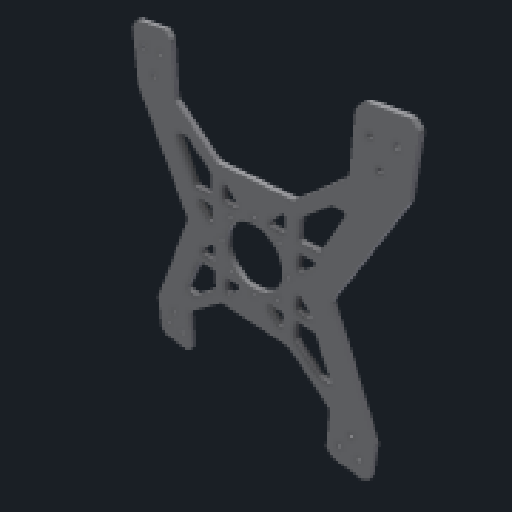
# Autodesk Inventor part: Root
Saved by Autodesk Inventor 2025.2 (Build 292293000, 293)
## iProperties
Created: 2020-05-07
Part Number: Root
Material: Generic
Document SubType Name: Sheet Metal
Designer: valer
Density: 1 g/cm^3
Sheet Metal Rule: Default
Appearance: Default
Author: valer
Autodesk Inventor part; units mm, degrees
ref_plane "YZ Plane" through (0, 0, 0) normal (1, 0, 0) x (0, 1, 0)
ref_plane "XZ Plane" through (0, 0, 0) normal (0, 1, 0) x (-1, 0, 0)
ref_plane "XY Plane" through (0, 0, 0) normal (0, 0, 1) x (1, 0, 0)
sketch "Base" plane through (0, 0, 0) normal (0, 0, 1) x (1, 0, 0)
  circle A0 centre (-56.25, 0) radius 2.75 construction
  circle A1 centre (0, -56.25) radius 2.75 construction
  circle A2 centre (0, 56.25) radius 2.75 construction
  circle A3 centre (39.7748, -39.7748) radius 2.75 construction
  circle A4 centre (-39.7748, 39.7748) radius 2.75 construction
  circle A5 centre (-39.7748, -39.7748) radius 2.75 construction
  circle A6 centre (39.7748, 39.7748) radius 2.75 construction
  circle A7 centre (56.25, 0) radius 2.75 construction
  circle A8 centre (0, 0) radius 45 construction
  circle A9 centre (0, 0) radius 61
  line L0 (-220, -170) -> (220, -170) construction
  line L1 (220, -170) -> (220, 210) construction
  line L2 (220, 210) -> (-220, 210) construction
  line L3 (-220, 210) -> (-220, -170) construction
  line L4 (0, -294) -> (0, 294) construction
  line L5 (-308, 0) -> (308, 0) construction
  line L6 (-220, 210) -> (-150, 210)
  line L7 (-150, 210) -> (-150, 130)
  line L8 (-150, 130) -> (-220, 130)
  line L9 (-220, 130) -> (-220, 210)
  line L10 (60, -103.923) -> (-60, -103.923)
  line L11 (-60, -103.923) -> (-120, 0)
  line L12 (-120, 0) -> (-60, 103.923)
  line L13 (-60, 103.923) -> (60, 103.923)
  line L14 (60, 103.923) -> (120, 0)
  line L15 (120, 0) -> (60, -103.923)
  line L16 (-120, 0) -> (-220, 130)
  line L17 (-150, 130) -> (-60, 103.923)
  line L18 (220, 210) -> (150, 210)
  line L19 (150, 210) -> (150, 130)
  line L20 (150, 130) -> (220, 130)
  line L21 (220, 130) -> (220, 210)
  line L22 (120, 0) -> (220, 130)
  line L23 (150, 130) -> (60, 103.923)
  line L24 (-220, -210) -> (-150, -210)
  line L25 (-150, -210) -> (-150, -130)
  line L26 (-150, -130) -> (-220, -170)
  line L27 (-220, -170) -> (-220, -210)
  line L28 (-120, 0) -> (-220, -170)
  line L29 (-150, -130) -> (-60, -103.923)
  line L30 (220, -170) -> (220, -210)
  line L31 (220, -210) -> (150, -210)
  line L32 (150, -210) -> (150, -130)
  line L33 (150, -130) -> (220, -170)
  line L34 (120, 0) -> (220, -170)
  line L35 (150, -130) -> (60, -103.923)
  circle A10 centre (0, 0) radius 46.5
  circle A11 centre (-56.25, 0) radius 2.25
  circle A12 centre (-39.7748, -39.7748) radius 2.25
  circle A13 centre (0, -56.25) radius 2.25
  circle A14 centre (39.7748, -39.7748) radius 2.25
  circle A15 centre (56.25, 0) radius 2.25
  circle A16 centre (39.7748, 39.7748) radius 2.25
  circle A17 centre (0, 56.25) radius 2.25
  circle A18 centre (-39.7748, 39.7748) radius 2.25
  point P0 (0, 0)
  point P1 (0, -170)
  dimension "d83" = 440
  dimension "d84" = 170
  dimension "d85" = 210
  dimension "d88" = 120
  dimension "d89" = 80
  dimension "d90" = 70
  dimension "d91" = 1.5
  dimension "d92" = 4.5
  measures "d83" distance of L0.start L0.end
  measures "d84" distance between parallel lines of L0 L5
  measures "d85" distance between parallel lines of L2 L5
  measures "d88" distance of L10.start L10.end
  measures "d89" distance between parallel lines of L2 L8
  measures "d90" distance between parallel lines of L7 L9
  measures "d91" radial gap between concentric circles of A10 A8
  measures "d92" diameter of A11
extrude "Plate1" add sketch "Base" against normal blind 8.4667 contours A9 | L6 L7 L8 L9 | L8 L17 L12 L16 | L12 L13 L14 L15 L10 L11 | L11 L29 L26 L28 | L26 L25 L24 L27 | L23 L20 L22 L14 | L15 L34 L33 L35 | L19 L18 L21 L20 | L33 L30 L31 L32
sketch "LegMountHoles" plane through (0, 0, -8.4667) normal (0, 0, -1) x (-1, 0, 0)
  line L0 (-120, 0) -> (-220, 130) construction
  line L1 (-150, 130) -> (-220, 130) construction
  line L2 (-220, 210) -> (-150, 210) construction
  line L3 (-185, 210) -> (-185, 130) construction
  line L4 (-170, 180) -> (-200, 180) construction
  circle A0 centre (-170, 180) radius 3
  circle A1 centre (-200, 180) radius 3
  circle A2 centre (-185, 150) radius 3
  line L5 (308, 0) -> (-308, 0) construction
  line L6 (0, -298) -> (0, 318) construction
  circle A3 centre (170, 180) radius 3
  circle A4 centre (200, 180) radius 3
  circle A5 centre (185, 150) radius 3
  circle A6 centre (-170, -180) radius 3
  circle A7 centre (-200, -180) radius 3
  circle A8 centre (-185, -150) radius 3
  circle A9 centre (170, -180) radius 3
  circle A10 centre (200, -180) radius 3
  circle A11 centre (185, -150) radius 3
  point P0 (0, 0)
  point P1 (-185, 180)
  dimension "d93" = 6
  dimension "d94" = 30
  dimension "d95" = 30
  dimension "d96" = 30
  constraints: 12 centre point, 9 symmetric about line, 6 end point, 3 midpoint, 2 coincident, 2 equal radius, 2 horizontal, 2 point on line, 9 other
  measures "d93" diameter of A0
  measures "d94" distance of L4.start L4.end
  measures "d95" distance from line of L4 A2.centre
  measures "d96" distance between parallel lines of L2 L4
extrude "LegMountHolesFeature" cut sketch "LegMountHoles" against normal blind 8.4667
sketch "StructureHoles" plane through (0, 0, -8.4667) normal (0, 0, -1) x (-1, 0, 0)
  line L0 (70.2991, 86.0845) -> (112.8625, 98.417)
  line L1 (112.8625, 98.417) -> (132.8625, 98.417)
  line L2 (132.8625, 98.417) -> (100.2991, 56.0845)
  line L3 (100.2991, 56.0845) -> (70.2991, 56.0845)
  line L4 (70.2991, 56.0845) -> (70.2991, 86.0845)
  line L5 (60, 103.923) -> (150, 130) projected
  line L6 (220, 130) -> (120, 0) construction
  line L7 (150, 210) -> (220, 210) projected
  line L8 (-60, 103.923) -> (60, 103.923) projected
  line L9 (60, 103.923) -> (120, 0) construction
  line L10 (50.2991, 86.0845) -> (50.2991, 56.0845)
  line L11 (50.2991, 56.0845) -> (20.2991, 56.0845)
  line L12 (20.2991, 56.0845) -> (50.2991, 86.0845)
  line L13 (70.2991, 86.0845) -> (50.2991, 86.0845) construction
  line L14 (308, 0) -> (-308, 0) construction
  line L15 (0, -298) -> (0, 318) construction
  line L16 (-70.2991, 86.0845) -> (-112.8625, 98.417)
  line L17 (-112.8625, 98.417) -> (-132.8625, 98.417)
  line L18 (-132.8625, 98.417) -> (-100.2991, 56.0845)
  line L19 (-100.2991, 56.0845) -> (-70.2991, 56.0845)
  line L20 (-70.2991, 56.0845) -> (-70.2991, 86.0845)
  line L21 (-50.2991, 86.0845) -> (-50.2991, 56.0845)
  line L22 (-50.2991, 56.0845) -> (-20.2991, 56.0845)
  line L23 (-20.2991, 56.0845) -> (-50.2991, 86.0845)
  line L24 (70.2991, -86.0845) -> (112.8625, -98.417)
  line L25 (112.8625, -98.417) -> (132.8625, -98.417)
  line L26 (132.8625, -98.417) -> (100.2991, -56.0845)
  line L27 (100.2991, -56.0845) -> (70.2991, -56.0845)
  line L28 (70.2991, -56.0845) -> (70.2991, -86.0845)
  line L29 (50.2991, -86.0845) -> (50.2991, -56.0845)
  line L30 (50.2991, -56.0845) -> (20.2991, -56.0845)
  line L31 (20.2991, -56.0845) -> (50.2991, -86.0845)
  line L32 (-132.8625, -98.417) -> (-100.2991, -56.0845)
  line L33 (-112.8625, -98.417) -> (-132.8625, -98.417)
  line L34 (-70.2991, -86.0845) -> (-112.8625, -98.417)
  line L35 (-70.2991, -56.0845) -> (-70.2991, -86.0845)
  line L36 (-100.2991, -56.0845) -> (-70.2991, -56.0845)
  line L37 (-50.2991, -86.0845) -> (-50.2991, -56.0845)
  line L38 (-20.2991, -56.0845) -> (-50.2991, -86.0845)
  line L39 (-50.2991, -56.0845) -> (-20.2991, -56.0845)
  line L40 (100.2991, 41.0845) -> (70.2991, 11.0845)
  line L41 (70.2991, 11.0845) -> (70.2991, 41.0845)
  line L42 (70.2991, 41.0845) -> (100.2991, 41.0845)
  line L43 (100.2991, 56.0845) -> (100.2991, 41.0845) construction
  line L44 (100.2991, -41.0845) -> (70.2991, -11.0845)
  line L45 (70.2991, -11.0845) -> (70.2991, -41.0845)
  line L46 (70.2991, -41.0845) -> (100.2991, -41.0845)
  line L47 (-100.2991, 41.0845) -> (-70.2991, 11.0845)
  line L48 (-70.2991, 11.0845) -> (-70.2991, 41.0845)
  line L49 (-70.2991, 41.0845) -> (-100.2991, 41.0845)
  line L50 (-100.2991, -41.0845) -> (-70.2991, -11.0845)
  line L51 (-70.2991, -41.0845) -> (-100.2991, -41.0845)
  line L52 (-70.2991, -11.0845) -> (-70.2991, -41.0845)
  point P0 (0, 0)
  point P1 (85.2991, 41.0845)
  dimension "d99" = 20
  dimension "d100" = 20
  dimension "d101" = 30
  dimension "d102" = 30
  dimension "d103" = 20
  dimension "d106" = 15
  constraints: 94 end point, 33 symmetric about line, 5 parallel, 4 perpendicular, 2 collinear, 2 equal length, 1 horizontal, 1 midpoint, 1 point on line, 1 vertical
  measures "d99" distance between parallel lines of L5 L0
  measures "d100" distance of L0.end L1.end
  measures "d101" distance of L3.end L0.start
  measures "d102" distance of L2.end L3.end
  measures "d103" distance of L0.start L10.start
  measures "d106" distance from line of point (85.299, 41.085) L3
extrude "StructureHolesFeature" cut sketch "StructureHoles" against normal blind 8.4667
fillet "InsideFilletsFeature" radius 4 44 edges at (-132.8625, 98.417, -4.2333) (-112.8625, 98.417, -4.2333) (-70.2991, 86.0845, -4.2333) (-70.2991, 56.0845, -4.2333) (-100.2991, 56.0845, -4.2333) (112.8625, 98.417, -4.2333) (132.8625, 98.417, -4.2333) (100.2991, 56.0845, -4.2333) (70.2991, 86.0845, -4.2333) (70.2991, 56.0845, -4.2333) (50.2991, 56.0845, -4.2333) (50.2991, 86.0845, -4.2333) (20.2991, 56.0845, -4.2333) (-50.2991, 86.0845, -4.2333) (-20.2991, 56.0845, -4.2333) (-50.2991, 56.0845, -4.2333) (-70.2991, 41.0845, -4.2333) (-100.2991, 41.0845, -4.2333) (-70.2991, 11.0845, -4.2333) (100.2991, 41.0845, -4.2333) (70.2991, 41.0845, -4.2333) (70.2991, 11.0845, -4.2333) (70.2991, -11.0845, -4.2333) (100.2991, -41.0845, -4.2333) (70.2991, -41.0845, -4.2333) (-100.2991, -41.0845, -4.2333) (-70.2991, -41.0845, -4.2333) (-70.2991, -11.0845, -4.2333) (-20.2991, -56.0845, -4.2333) (-50.2991, -86.0845, -4.2333) (-50.2991, -56.0845, -4.2333) (50.2991, -86.0845, -4.2333) (20.2991, -56.0845, -4.2333) (50.2991, -56.0845, -4.2333) (-132.8625, -98.417, -4.2333) (-100.2991, -56.0845, -4.2333) (-70.2991, -56.0845, -4.2333) (-70.2991, -86.0845, -4.2333) (70.2991, -56.0845, -4.2333) (70.2991, -86.0845, -4.2333) (112.8625, -98.417, -4.2333) (132.8625, -98.417, -4.2333) (100.2991, -56.0845, -4.2333) (-112.8625, -98.417, -4.2333)
chamfer "OutsideChamfersFeature" distance 10 angle 45 8 edges at (-220, -210, -4.2333) (-150, -210, -4.2333) (150, -210, -4.2333) (220, -210, -4.2333) (-220, 210, -4.2333) (-150, 210, -4.2333) (150, 210, -4.2333) (220, 210, -4.2333)
fillet "OutsideFilletsFeature" radius 8 30 edges at (60, 103.923, -4.2333) (150, 130, -4.2333) (150, 200, -4.2333) (160, 210, -4.2333) (210, 210, -4.2333) (220, 200, -4.2333) (220, 130, -4.2333) (120, 0, -4.2333) (220, -170, -4.2333) (220, -200, -4.2333) (210, -210, -4.2333) (160, -210, -4.2333) (150, -200, -4.2333) (150, -130, -4.2333) (60, -103.923, -4.2333) (-60, -103.923, -4.2333) (-160, -210, -4.2333) (-150, -200, -4.2333) (-210, -210, -4.2333) (-220, -200, -4.2333) (-220, -170, -4.2333) (-150, -130, -4.2333) (-120, 0, -4.2333) (-220, 130, -4.2333) (-220, 200, -4.2333) (-210, 210, -4.2333) (-160, 210, -4.2333) (-150, 200, -4.2333) (-60, 103.923, -4.2333) (-150, 130, -4.2333)
equation "\"d97\" = Thickness"
equation "\"d104\" = Thickness"
equation "\"d33\" = Thickness"
equation "\"BendRadius\" = Thickness"
equation "\"BendReliefWidth\" = Thickness"
equation "\"BendReliefDepth\" = 0.5 * Thickness"
equation "\"CornerReliefSize\" = 4 * Thickness"
equation "\"MinimumRemnant\" = 2 * Thickness"
equation "\"TransitionRadius\" = BendRadius"
equation "\"JacobiRadiusSize\" = BendRadius"
equation "\"GapSize\" = Thickness"
equation "\"Thickness\" = 8.466667"
body "Solid1"
